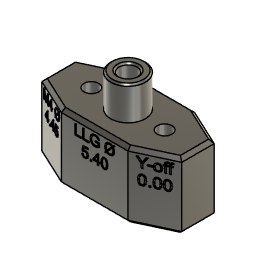
Lightcrafter_LLG_3mm_adapter (Autodesk Fusion 360 design; units mm, degrees)
Autodesk Fusion 360 part; units mm, degrees
sketch "Base" plane through (0, 0, 0) normal (0, 0, 1) x (1, 0, 0)
  line L0 (-21, 0) -> (-21, 4.8706)
  line L1 (-21, 4.8706) -> (-10, 10)
  line L2 (-10, 10) -> (0, 10)
  line L3 (0, 0) -> (-11, 0) construction
  line L4 (-11, 0) -> (-21, 0) construction
  circle A0 centre (-11, 0) radius 2.225
  line L5 (0, 0) -> (0, 10) construction
  line L6 (21, 4.8706) -> (10, 10)
  line L7 (10, 10) -> (0, 10)
  line L8 (21, 0) -> (21, 4.8706)
  circle A1 centre (11, 0) radius 2.225
  line L9 (21, 0) -> (21, -4.8706)
  line L10 (21, -4.8706) -> (10, -10)
  line L11 (10, -10) -> (0, -10)
  line L12 (-10, -10) -> (0, -10)
  line L13 (-21, -4.8706) -> (-10, -10)
  line L14 (-21, 0) -> (-21, -4.8706)
  line L15 (0, 0) -> (0, -0.001) construction
  circle A2 centre (0, -0.001) radius 2.7
  circle A3 centre (0, -0.001) radius 6
  dimension "d4" = 4.45
  dimension "d5" = 10
  dimension "d6" = 11
  dimension "d7" = 10
  dimension "d9" = 115
  dimension "d10" = 10
  dimension "d42" = 0.001
  dimension "d43" = 5.4
  dimension "d53" = 12
  constraint perpendicular L0 L2
  constraint perpendicular L0 L4
  constraint coincident L3.end L4.start
  constraint horizontal L2
  constraint perpendicular L3 L5
  constraint coincident L2.end L5.end
  constraint symmetric L0.start L5 L8.start
  constraint symmetric L0.end L5 L6.start
  constraint symmetric L1.end L5 L6.end
  constraint symmetric L2.end L5 L7.end
  constraint symmetric A0 L5 A1
  constraint symmetric L0.start L3 L4.end
  constraint symmetric L0.end L3 L13.start
  constraint symmetric L1.end L3 L12.start
  constraint symmetric L2.end L3 L11.end
  constraint symmetric L3 L6.end L10.end
  constraint symmetric L3 L6.start L9.end
  constraint symmetric L3 L2.end L11.end
  constraint symmetric L3 L8.start L9.start
  constraint coincident L0.start L4.end
  constraint coincident L3.start L5.start
  constraint perpendicular L3 L15
  constraint coincident L15.end A2.centre
  constraint concentric A2 A3
  measures "d4" diameter of A0
  measures "d5" distance of L3.start L2.end
  measures "d6" distance of L3.start L3.end
  measures "d7" distance of L0.start L3.end
  measures "d9" angle of L0 L1
  measures "d10" distance of L1.end L2.end
  measures "d42" distance of L3.start L15.end
  measures "d43" diameter of A2
  measures "d53" diameter of A3
extrude "Extrude1" add sketch "Base" along normal blind 10 contours L0 L1 L2 L6 L7 L8 L9 L10 L11 L12 L13 L14 | A3 makes body 1
extrude "Extrude2" add sketch "Base" along normal blind 20 separate body contours A2 makes body 2
shell "Shell1" thickness 2.5 outward yes removed faces 2 at (0.4274, -0.9303, 20) at (0.4274, -0.9303, 0) on bodies 2
combine "Combine1" operation add target body 1 tool bodies 2
extrude "Extrude3" add sketch "Base" against normal blind 10 contours L0 L1 L2 L6 L7 L8 L9 L10 L11 L12 L13 L14 bodies 1
chamfer "Chamfer1" distance 1 angle 45 8 edges at (21, 0, 10) (15.5, -7.4353, 10) (0, -10, 10) (-15.5, -7.4353, 10) (-21, 0, 10) (-15.5, 7.4353, 10) (0, 10, 10) (15.5, 7.4353, 10) 1 faces at (18.4083, 0, -10) on bodies 1
chamfer "Chamfer1" distance 0.5 angle 45 1 faces at (4.3473, 0.2573, 20) on bodies 1
chamfer "Chamfer1" distance 3 angle 45 1 edges at (-2.5173, 0.9754, 0) on bodies 1
sketch "Label_LLG" plane through (0, -10, 0) normal (0, -1, 0) x (1, 0, 0)
  line L0 (-10, -9) -> (10, -9)
  line L1 (10, -9) -> (10, 9)
  line L2 (10, 9) -> (-10, 9)
  line L3 (-10, 9) -> (-10, -9)
  line L4 (-10, 4.5) -> (10, 4.5) construction
  line L5 (10, 4.5) -> (10, 9) construction
  line L6 (10, 9) -> (-10, 9) construction
  line L7 (-10, 9) -> (-10, 4.5) construction
  line L8 (-10, 0) -> (10, 0) construction
  line L9 (10, 0) -> (10, 4.5) construction
  line L10 (10, 4.5) -> (-10, 4.5) construction
  line L11 (-10, 4.5) -> (-10, 0) construction
  dimension "d35" = 3
  dimension "d36" = 3
  text T0 "LLG Ø" font "Arial" height 3 align centre middle in box 20 x 4.5 at (-10, 4.5) x (1, 0) y (0, 1) spacing 1 kerned
  text T1 "5.40" font "Arial" height 3 align centre middle in box 20 x 4.5 at (-10, 0) x (1, 0) y (0, 1) spacing 1 kerned
  constraint coincident L2.end
  constraint coincident L1
  constraint coincident L1.end
  constraint coincident origin L8
  constraint equal L5 L9
sketch "Label_M4" plane through (-5.6163, -12.0442, 0) normal (-0.422618, -0.906308, 0) x (0.906308, -0.422618, 0)
  line L0 (-16.9741, -9) -> (-4.8369, -9)
  line L1 (-4.8369, -9) -> (-4.8369, 9)
  line L2 (-4.8369, 9) -> (-16.9741, 9)
  line L3 (-16.9741, 9) -> (-16.9741, -9)
  line L4 (-16.9741, 4.5) -> (-4.8369, 4.5) construction
  line L5 (-4.8369, 4.5) -> (-4.8369, 9) construction
  line L6 (-4.8369, 9) -> (-16.9741, 9) construction
  line L7 (-16.9741, 9) -> (-16.9741, 4.5) construction
  line L8 (-16.9741, 0) -> (-4.8369, 0) construction
  line L9 (-4.8369, 0) -> (-4.8369, 4.5) construction
  line L10 (-4.8369, 4.5) -> (-16.9741, 4.5) construction
  line L11 (-16.9741, 4.5) -> (-16.9741, 0) construction
  line L12 (0, 0) -> (-4.8369, 0) construction
  point P0 (-4.8369, 9)
  point P1 (-16.9741, 0)
  dimension "d37" = 3
  dimension "d38" = 3
  text T0 "M4 Ø" font "Arial" height 3 align centre middle in box 12.1372 x 4.5 at (-16.9741, 4.5) x (1, 0) y (0, 1) spacing 1 kerned
  text T1 "4.45" font "Arial" height 3 align centre middle in box 12.1372 x 4.5 at (-16.9741, 0) x (1, 0) y (0, 1) spacing 1 kerned
  constraint coincident L1
  constraint coincident L2.end
  constraint equal L5 L9
  constraint coincident L12.start origin
  constraint perpendicular L1 L12
  constraint coincident L1 L8.end
  constraint coincident L8.end
sketch "Labe_yoff" plane through (5.6163, -12.0442, 0) normal (0.422618, -0.906308, 0) x (0.906308, 0.422618, 0)
  line L0 (4.8369, -9) -> (16.9741, -9)
  line L1 (16.9741, -9) -> (16.9741, 9)
  line L2 (16.9741, 9) -> (4.8369, 9)
  line L3 (4.8369, 9) -> (4.8369, -9)
  line L4 (4.8369, 4.5) -> (16.9741, 4.5) construction
  line L5 (16.9741, 4.5) -> (16.9741, 9) construction
  line L6 (16.9741, 9) -> (4.8369, 9) construction
  line L7 (4.8369, 9) -> (4.8369, 4.5) construction
  line L8 (4.8369, 0) -> (16.9741, 0) construction
  line L9 (16.9741, 0) -> (16.9741, 4.5) construction
  line L10 (16.9741, 4.5) -> (4.8369, 4.5) construction
  line L11 (4.8369, 4.5) -> (4.8369, 0) construction
  line L12 (0, 0) -> (16.9741, 0) construction
  dimension "d45" = 3
  dimension "d46" = 3
  text T0 "Y-off" font "Arial" height 3 align centre middle in box 12.1372 x 4.5 at (4.8369, 4.5) x (1, 0) y (0, 1) spacing 1 kerned
  text T1 "0.00" font "Arial" height 3 align centre middle in box 12.1372 x 4.5 at (4.8369, 0) x (1, 0) y (0, 1) spacing 1 kerned
  constraint coincident L2.end
  constraint coincident L1.end
  constraint equal L5 L9
  constraint coincident L12.start origin
  constraint perpendicular L1 L12
  constraint coincident L1 L8.end
  constraint collinear L8 L12
sketch "Label_version" plane through (0, 10, 0) normal (0, 1, 0) x (-1, 0, 0)
  line L0 (-10, -9) -> (10, -9)
  line L1 (10, -9) -> (10, 9)
  line L2 (10, 9) -> (-10, 9)
  line L3 (-10, 9) -> (-10, -9)
  line L4 (-10, -9) -> (10, -9) construction
  line L5 (10, -9) -> (10, 9) construction
  line L6 (10, 9) -> (-10, 9) construction
  line L7 (-10, 9) -> (-10, -9) construction
  dimension "d47" = 3
  text T0 "v14" font "Arial" height 3 align centre middle in box 20 x 18 at (-10, -9) x (1, 0) y (0, 1) spacing 1 kerned
  constraint coincident L2.end
  constraint coincident L0.end
extrude "Extrude6" cut sketch "Label_M4" sketch "Label_LLG" sketch "Labe_yoff" against normal blind 0.5 text T0 T1 of sketch 2 text T0 T1 of sketch 3 text T0 T1 bodies 1
extrude "Extrude7" cut sketch "Label_version" against normal blind 0.5 text T0 bodies 1
equation "LLG_dia = LLG_dia_base + LLG_dia_tol"
equation "LLG_dia_base = 4.9 mm"
equation "d4 = M4_dia"
equation "LLG_dia_tol = 0.5 mm"
equation "M4_dia = M4_dia_base + M4_dia_tol"
equation "M4_dia_base = 4.0 mm"
equation "M4_dia_tol = 0.45 mm"
equation "Y_offset = 0.001 mm"
equation "d42 = Y_offset"
equation "d43 = LLG_dia"
